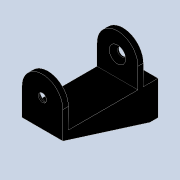
# Autodesk Inventor part: X Axis Drag Chain Mount Moble
Saved by Autodesk Inventor 2022 (Build 260153000, 153)
## iProperties
Created: 2021-10-30
Part Number: X Axis Drag Chain Mount Moble
Material: Generic
Document SubType Name: Modeling
Designer: Coy
Density: 1 g/cm^3
Appearance: Anodized - Black
Author: Coy
Autodesk Inventor part; units mm, degrees
ref_plane "YZ Plane" through (0, 0, 0) normal (1, 0, 0) x (0, 1, 0)
ref_plane "XZ Plane" through (0, 0, 0) normal (0, 1, 0) x (-1, 0, 0)
ref_plane "XY Plane" through (0, 0, 0) normal (0, 0, 1) x (1, 0, 0)
sketch "Sketch1" plane through (0, 0, 0) normal (0, 0, 1) x (1, 0, 0)
  line L0 (0, 0) -> (-30, 0)
  line L1 (-30, 0) -> (-30, 20)
  line L2 (-30, 20) -> (0, 20)
  line L3 (0, 20) -> (0, 0)
  line L4 (0, 20) -> (-30, 20)
  line L5 (-30, 20) -> (-30, 55)
  line L6 (-30, 55) -> (0, 55)
  line L7 (0, 55) -> (0, 20)
  line L8 (-20, 15) -> (-10, 15) construction
  line L9 (-10, 15) -> (-10, 5) construction
  line L10 (-10, 5) -> (-20, 5) construction
  line L11 (-20, 5) -> (-20, 15) construction
  line L12 (-15, 15) -> (-15, 20) construction
  line L13 (-20, 10) -> (-30, 10) construction
  circle A0 centre (-20, 15) radius 2.6
  circle A1 centre (-10, 5) radius 2.6
  dimension "d0" = 30
  dimension "d1" = 20
  dimension "d2" = 30
  dimension "d3" = 35
  dimension "d4" = 10
  dimension "d5" = 10
  dimension "d6" = 5.2
  dimension "d8" = 5.2
  constraints: 28 end point, 6 parallel, 5 perpendicular, 4 midpoint, 3 horizontal, 2 centre point, 2 coincident
  measures "d0" distance of L1.end L2.end
  measures "d1" distance of L0.end L1.end
  measures "d2" distance of L5.end L6.end
  measures "d3" distance of L4.end L5.end
  measures "d4" distance of L8.start L8.end
  measures "d5" distance of L10.end L8.start
  measures "d6" diameter of A0
  measures "d8" diameter of A1
extrude "Extrusion1" add sketch "Sketch1" along normal blind 14.75
sketch "Sketch2" plane through (0, 0, 14.75) normal (0, 0, 1) x (1, 0, 0)
  line L0 (0, 0) -> (0, 55) projected
  line L1 (0, 20) -> (-30, 20)
  line L2 (-30, 20) -> (-30, 25)
  line L3 (-30, 25) -> (0, 25)
  line L4 (0, 25) -> (0, 20)
  line L5 (-30, 0) -> (0, 0) projected
  line L6 (-30, 55) -> (-30, 0) projected
  point P0 (0, 25)
  dimension "d14" = 5
  dimension "d15" = 20
  constraints: 8 end point, 2 parallel, 1 collinear, 1 horizontal, 1 perpendicular, 1 point on line
  measures "d14" distance of L1.end L2.end
  measures "d15" distance between parallel lines of L5 L1
extrude "Extrusion2" add sketch "Sketch2" along normal blind 51 contours L1 L2 L3 L0
sketch "Sketch3" plane through (0, 0, 65.75) normal (0, 0, 1) x (1, 0, 0)
  line L0 (-30, 25) -> (0, 25) projected
  line L1 (0, 25) -> (0, 55) projected
  line L2 (0, 55) -> (-30, 55) projected
  line L3 (-30, 55) -> (-30, 25) projected
  line L4 (-30, 20) -> (0, 20) projected
  line L5 (0, 20) -> (0, 25) projected
  line L6 (0, 25) -> (-30, 25) projected
  line L7 (-30, 25) -> (-30, 20) projected
  line L8 (-30, 0) -> (0, 0) projected
  line L9 (0, 0) -> (0, 20) projected
  line L10 (0, 20) -> (-30, 20) projected
  line L11 (-30, 20) -> (-30, 0) projected
  point P0 (0, 25)
extrude "Extrusion3" add sketch "Sketch3" along normal blind 4 contours L3 L2 L1 L0 | L0 L5 L4 L7
sketch "Sketch4" plane through (0, 0, 0) normal (1, 0, 0) x (0, 0, -1)
  line L0 (-14.75, 55) -> (-14.75, 0) projected
  line L1 (-14.75, 20) -> (-6, 20)
  line L2 (-6, 20) -> (-6, 0)
  line L3 (-6, 0) -> (-14.75, 0)
  line L4 (-14.75, 0) -> (-14.75, 20)
  line L5 (0, 55) -> (-14.75, 55) projected
  line L6 (0, 55) -> (-10.75, 55)
  line L7 (-10.75, 55) -> (-10.75, 25)
  line L8 (-10.75, 25) -> (0, 25)
  line L9 (0, 25) -> (0, 55)
  line L10 (-14.75, 25) -> (-14.75, 55) projected
  line L11 (0, 0) -> (0, 55) projected
  point P0 (-14.75, 0)
  dimension "d21" = 20
  dimension "d22" = 30
  dimension "d23" = 4
  dimension "d50" = 6
  constraints: 16 end point, 4 parallel, 2 horizontal, 2 perpendicular
  measures "d21" distance of L1.end L2.end
  measures "d22" distance of L6.end L7.end
  measures "d23" distance between parallel lines of L10 L7
  measures "d50" distance between parallel lines of L11 L2
extrude "Extrusion4" cut sketch "Sketch4" against normal through all
sketch "Sketch6" plane through (0, 0, 6) normal (0, 0, 1) x (1, 0, 0)
  line L0 (-30, 20) -> (0, 20) projected
  line L1 (-30, 0) -> (0, 0) projected
  line L2 (0, 20) -> (-4, 20)
  line L3 (-4, 20) -> (-4, 0)
  line L4 (-4, 0) -> (0, 0)
  line L5 (0, 0) -> (0, 20)
  line L6 (-30, 55) -> (-30, 20) projected
  line L7 (-30, 20) -> (-26, 20)
  line L8 (-26, 20) -> (-26, 0)
  line L9 (-26, 0) -> (-30, 0)
  line L10 (-30, 0) -> (-30, 20)
  point P0 (-26, 0)
  dimension "d33" = 4
  dimension "d34" = 4
  constraints: 16 end point, 4 parallel, 2 horizontal, 2 perpendicular, 2 point on line
  measures "d33" distance of L4.end L3.end
  measures "d34" distance of L8.end L9.end
extrude "Extrusion6" add sketch "Sketch6" along normal up to surface (63.75 mm away) contours L0 L8 L1 L10 | L0 L5 L1 L3
chamfer "Chamfer2" distance 63.75 distance2 20 1 edges at (-2, 0, 69.75) measured on face at (-1.3333, 0, 25.25)
chamfer "Chamfer3" distance 63.75 distance2 20 1 edges at (-28, 0, 69.75) measured on face at (-28.6667, 0, 25.25)
fillet "Fillet1" radius 15 4 edges at (-30, 55, 67.75) (0, 55, 67.75) (-30, 55, 12.75) (0, 55, 12.75)
sketch "Sketch7" plane through (0, 0, 69.75) normal (0, 0, 1) x (1, 0, 0)
  arc A0 (0, 40) -> (-30, 40) centre (-15, 40) ccw projected
  circle A1 centre (-15, 40) radius 3
  point P0 (0, 0)
  dimension "d44" = 6
  constraints: 1 centre point, 1 coincident
  measures "d44" diameter of A1
extrude "Extrusion7" cut sketch "Sketch7" against normal through all
chamfer "Chamfer4" distance 3 angle 45 2 edges at (-18, 40, 14.75) (-18, 40, 65.75)
equation "\"d8\" = d6"
body "Solid1"
